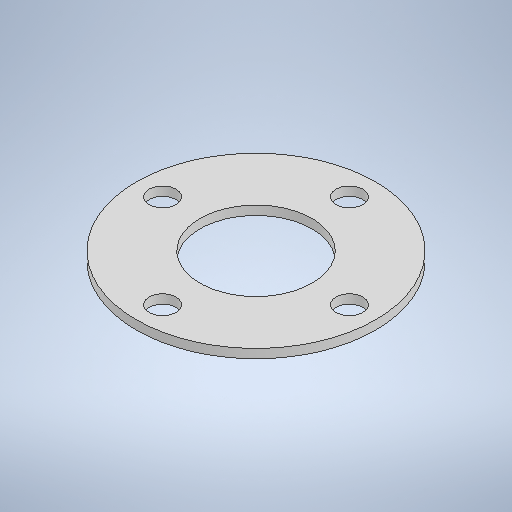
# Autodesk Inventor part: SLM 1431 FDS flange DN90
Saved by Autodesk Inventor 2025.4 (Build 294407000, 407)
## iProperties
Created: 2025-02-13
Part Number: SLM 1431 FDS flange DN90
Material: Steel
Document SubType Name: Sheet Metal
Designer: admin
Mass: 1559.54 g
Surface Area: 600.468 cm^2
Volume: 198.668 cm^3
Density: 7.85 g/cm^3
Flat Pattern Width: 16 cm
Flat Pattern Length: 16 cm
Flat Pattern Area: 256 cm^2
Sheet Metal Rule: AISI304 4mm Die 32
Sheet Metal Width: 160,000 mm
Sheet Metal Length: 160,000 mm
Sheet Metal Area: 25600,000 mm^2
Appearance: Default
Author: pokla
Autodesk Inventor part; units mm, degrees
ref_plane "YZ Plane" through (0, 0, 0) normal (1, 0, 0) x (0, 1, 0)
ref_plane "XZ Plane" through (0, 0, 0) normal (0, 1, 0) x (-1, 0, 0)
ref_plane "XY Plane" through (0, 0, 0) normal (0, 0, 1) x (1, 0, 0)
sketch "Sketch2" plane through (0, 0, 0) normal (0, 0, 1) x (1, 0, 0)
  circle A0 centre (0, 0) radius 37.5
  circle A1 centre (0, 0) radius 80
  circle A2 centre (0, 0) radius 62.5 construction
  circle A3 centre (0, 62.5) radius 9
  circle A4 centre (-62.5, 0) radius 9
  circle A5 centre (0, -62.5) radius 9
  circle A6 centre (62.5, 0) radius 9
  dimension "d29" = 125
  dimension "d25" = 75
  dimension "d27" = 160
  dimension "d30" = 18
  dimension "d33" = 360
  measures "d25" diameter of A0
  measures "d27" diameter of A1
  measures "d30" diameter of A3
extrude "Plate2" add sketch "Sketch2" along normal blind 6
equation "\"d14\" = Thickness"
equation "\"BendReliefWidth\" = Thickness"
equation "\"BendReliefDepth\" = 0.5 * Thickness"
equation "\"CornerReliefSize\" = 4 * Thickness"
equation "\"MinimumRemnant\" = 2 * Thickness"
equation "\"TransitionRadius\" = BendRadius"
equation "\"JacobiRadiusSize\" = BendRadius"
equation "\"GapSize\" = Thickness"
equation "\"Thickness\" = 6"
equation "\"BendRadius\" = 6"
body "Solid3"
